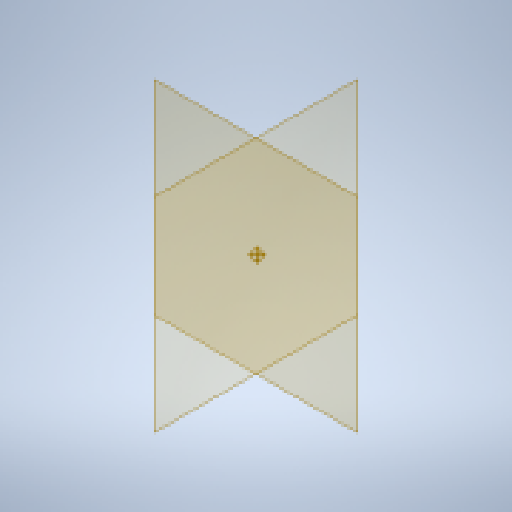
# Autodesk Inventor part: ArmSolenoidShaftBoundingBox
Saved by Autodesk Inventor 2023 (Build 270158000, 158)
## iProperties
Created: 2023-03-30
Part Number: ArmSolenoidShaftBoundingBox
Material: Generic
Document SubType Name: Modeling
Designer: LattePanda
Density: 1 g/cm^3
Appearance: Default
Author: LattePanda
Autodesk Inventor part; units mm, degrees
ref_plane "XZ Plane" through (0, 0, 0) normal (0, 1, 0) x (-1, 0, 0)
ref_plane "Work Plane1" through (-17.3808, -12.8161, -79.6267) normal (0, 0, 1) x (1, 0, 0)
sketch "Sketch2" plane through (-17.3808, -12.8161, -79.6267) normal (0, 0, 1) x (1, 0, 0)
  circle A0 centre (0, 0) radius 3.175 projected
  line L0 (2.7795, -1.5347) -> (0.0606, -3.1744)
  line L1 (0.0606, -3.1744) -> (-2.7188, -1.6397)
  line L2 (-2.7188, -1.6397) -> (-2.7795, 1.5347)
  line L3 (-2.7795, 1.5347) -> (-0.0606, 3.1744)
  line L4 (-0.0606, 3.1744) -> (2.7188, 1.6397)
  line L5 (2.7188, 1.6397) -> (2.7795, -1.5347)
  point P0 (17.3808, 12.8161)
  constraints: 12 end point, 1 coincident, 15 other
ref_plane "Work Plane2" through (-16.1743, -15.6151, -101.1913) normal (0, 0, -1) x (0, 1, 0)
extrude "Extrusion1" add sketch "Sketch2" against normal up to surface (21.5646 mm away) contours L5 L0 L1 L2 L3 L4
body "Solid1"
